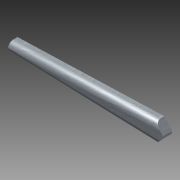
# Autodesk Inventor part: Thrust_Support
Saved by Autodesk Inventor 2011 SP1 (Build 150282100, 282)
## iProperties
Created: 2011-06-11
Part Number: Thrust_Support
Document SubType Name: Modeling
Designer: Andrew G. Meyer
Mass: 5.49048 g
Surface Area: 29.7174 cm^2
Volume: 5.49048 cm^3
Density: 1 g/cm^3
Author: Andrew G. Meyer
Autodesk Inventor part; units mm, degrees
ref_plane "YZ Plane" through (0, 0, 0) normal (1, 0, 0) x (0, 1, 0)
ref_plane "XZ Plane" through (0, 0, 0) normal (0, 1, 0) x (-1, 0, 0)
ref_plane "XY Plane" through (0, 0, 0) normal (0, 0, 1) x (1, 0, 0)
sketch "Sketch1" plane through (0, 0, 0) normal (0, 0, 1) x (1, 0, 0)
  line L0 (0, 0) -> (-6.35, 6.35)
  line L1 (-6.35, 6.35) -> (-103.1386, 3.175)
  line L2 (-103.1386, -3.175) -> (-6.35, -6.35)
  line L3 (-6.35, -6.35) -> (0, 0)
  arc A0 (-103.1386, 3.175) -> (-103.1386, -3.175) centre (0, 0) ccw
  line L4 (0, 0) -> (0.1245, 0) construction
  dimension "d1" = 6.35
  dimension "d3" = 6.35
  dimension "d10" = 135
  dimension "d11" = 103.1875
  constraints: 10 end point, 2 coincident, 2 equal length, 2 point on circle, 1 centre point, 1 horizontal, 1 perpendicular
  measures "d1" horizontal distance of point (0, 0) L0.end
  measures "d3" distance of L2.start L1.end
  measures "d10" angle of L4 L0
  measures "d11" radius of A0
extrude "Extrusion1" add sketch "Sketch1" along normal blind 6.35
fillet "Fillet2" radius 3.81 2 edges at (-54.7443, -4.7625, 6.35) (-54.7443, 4.7625, 6.35)
hole "Hole1" at (0, 0, 6.35) direction (0, 0, -1) diameter 3.175 depth 25.4 tip angle 118
body "Solid1"
